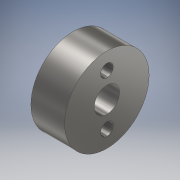
# Autodesk Inventor part: スリットカラー
Saved by Autodesk Inventor 2018 (Build 220112000, 112)
## iProperties
Created: 2019-04-22
Part Number: スリットカラー
Material: ステンレス鋼
Document SubType Name: Modeling
Designer: Eiji Nishizawa
Density: 8 g/cm^3
Appearance: 半つや出し
Author: Eiji Nishizawa
Autodesk Inventor part; units mm, degrees
ref_plane "YZ Plane" through (0, 0, 0) normal (1, 0, 0) x (0, 1, 0)
ref_plane "XZ Plane" through (0, 0, 0) normal (0, 1, 0) x (-1, 0, 0)
ref_plane "XY Plane" through (0, 0, 0) normal (0, 0, 1) x (1, 0, 0)
sketch "スケッチ1" plane through (0, 0, 0) normal (1, 0, 0) x (0, 1, 0)
  circle A0 centre (0, 0) radius 10
  circle A1 centre (0, 0) radius 3
  circle A2 centre (0, 6) radius 1.5
  circle A3 centre (0, -6) radius 1.5
  dimension "d0" = 20
  dimension "d1" = 6
  dimension "d2" = 9
  dimension "d3" = 3
  dimension "d4" = 3
  dimension "d5" = 6
  dimension "d6" = 6
  constraints: 4 centre point, 2 coincident
  measures "d0" diameter of A0
  measures "d1" diameter of A1
  measures "d3" diameter of A2
  measures "d4" diameter of A3
  measures "d5" distance of point (0, 0) A2.centre
  measures "d6" distance of point (0, 0) A3.centre
extrude "押し出し1" add sketch "スケッチ1" along normal blind 8
